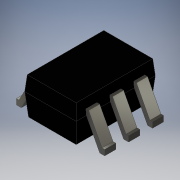
# Autodesk Inventor part: TI_DCK
Saved by Autodesk Inventor 2016 (Build 200138000, 138)
## iProperties
Created: 2016-09-01
Part Number: TI_DCK
Material: Generic
Document SubType Name: Modeling
Designer: jfixelle
Density: 1 g/cm^3
Appearance: Black
Author: jfixelle
Autodesk Inventor part; units mm, degrees
ref_plane "YZ Plane" through (0, 0, 0) normal (1, 0, 0) x (0, 1, 0)
ref_plane "XZ Plane" through (0, 0, 0) normal (0, 1, 0) x (-1, 0, 0)
ref_plane "XY Plane" through (0, 0, 0) normal (0, 0, 1) x (1, 0, 0)
sketch "Sketch1" plane through (0, 0, 0) normal (0, 1, 0) x (-1, 0, 0)
  line L0 (0.7, 1.075) -> (-0.7, 1.075)
  line L1 (-0.7, 1.075) -> (-0.7, -1.075)
  line L2 (-0.7, -1.075) -> (0.7, -1.075)
  line L3 (0.7, -1.075) -> (0.7, 1.075)
  point P0 (0, 0)
  dimension "d0" = 2.15
  dimension "d1" = 1.4
  dimension "d2" = 0.7
  dimension "d3" = 1.075
  constraints: 8 end point, 2 parallel, 1 horizontal, 1 perpendicular
  measures "d0" distance of L2.end L0.start
  measures "d1" distance of L1.end L2.end
  measures "d2" distance from line of point (0, 0) L3
  measures "d3" distance from line of point (0, 0) L2
extrude "Extrusion1" add sketch "Sketch1" along normal blind 1
chamfer "Chamfer1" distance 0.4 angle 5 1 edges at (0.7, 1, 0) measured on face at (0.7, 0.3333, 0.3583)
chamfer "Chamfer2" distance 0.4 angle 5 1 edges at (-0.0175, 1, 1.075) measured on face at (-0.2333, 0.5333, 1.075)
chamfer "Chamfer3" distance 0.4 angle 5 1 edges at (-0.0175, 1, -1.075) measured on face at (-0.2333, 0.5333, -1.075)
chamfer "Chamfer4" distance 0.4 angle 5 1 edges at (-0.7, 1, 0) measured on face at (-0.7, 0.2, -0.3583)
chamfer "Chamfer5" distance 0.6 angle 5 1 edges at (0.7, 0, 0) measured on face at (0.7, 0.2, 0.3583)
chamfer "Chamfer6" distance 0.6 angle 5 1 edges at (-0.0262, 0, -1.075) measured on face at (0.2159, 0.4, -1.075)
chamfer "Chamfer7" distance 0.6 angle 5 1 edges at (-0.7, 0, 0.0262) measured on face at (-0.7, 0.4, -0.3409)
chamfer "Chamfer8" distance 0.6 angle 5 1 edges at (0, 0, 1.075) measured on face at (0.2159, 0.3999, 1.075)
sketch "Sketch3" plane through (0, 0, 0) normal (0, 0, 1) x (1, 0, 0)
  line L0 (0.6067, 0.75) -> (0.6067, 0.6)
  line L1 (0.6067, 0.6) -> (0.7002, 0.6)
  line L2 (0.7002, 0.6) -> (1.0651, -0.1)
  line L3 (1.0651, -0.1) -> (1.2, -0.1)
  line L4 (1.2, -0.1) -> (1.2, 0.05)
  line L5 (1.2, 0.05) -> (1.1276, 0.05)
  line L6 (1.1276, 0.05) -> (0.7628, 0.75)
  line L7 (0.7628, 0.75) -> (0.6067, 0.75)
  line L8 (-0.6475, 0) -> (0.6475, 0) projected
  line L9 (-0.7, 0.6) -> (0.7, 0.6) projected
  line L10 (0, 0) -> (0, -0.004)
  dimension "d30" = 0.15
  dimension "d31" = 0.15
  dimension "d33" = 0.1
  dimension "d34" = 0
  dimension "d35" = 1.2
  constraints: 18 end point, 3 parallel, 3 perpendicular, 2 vertical
  measures "d30" distance between parallel lines of L3 L5
  measures "d31" distance between parallel lines of L1 L7
  measures "d33" distance between parallel lines of L3 L8
  measures "d34" distance between parallel lines of L9 L1
  measures "d35" distance between parallel lines of L4 L10
extrude "Extrusion2" add sketch "Sketch3" along normal mid plane 0.3
pattern_linear "Rectangular Pattern1" count 3 spacing 0.65 along (0, 0, 1) of "Extrusion2" first direction both ways yes
mirror "Mirror1" about plane through (0, 0, 0) normal (1, 0, 0) of "Extrusion2", "Rectangular Pattern1"
body "Solid1"
